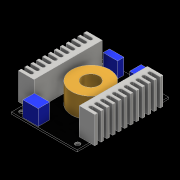
# Autodesk Inventor part: DROK_090483
Saved by Autodesk Inventor 2016 (Build 200138000, 138)
## iProperties
Created: 2016-05-04
Part Number: DROK_090483
Material: Generic
Document SubType Name: Modeling
Designer: CamB
Mass: 20.71 g
Surface Area: 169.365 cm^2
Volume: 20.71 cm^3
Density: 1 g/cm^3
Appearance: Default
Author: CamB
Autodesk Inventor part; units mm, degrees
ref_plane "YZ Plane" through (0, 0, 0) normal (1, 0, 0) x (0, 1, 0)
ref_plane "XZ Plane" through (0, 0, 0) normal (0, 1, 0) x (-1, 0, 0)
sketch "Sketch1" plane through (0, 0, 0) normal (0, 0, 1) x (1, 0, 0)
  line L0 (0, 0) -> (43, 0)
  line L1 (43, 0) -> (43, 60)
  line L2 (43, 60) -> (0, 60)
  line L3 (0, 60) -> (0, 0)
  dimension "d0" = 43
  dimension "d1" = 60
  constraints: 8 end point, 2 parallel, 1 horizontal, 1 perpendicular
  measures "d0" distance of L2.end L1.end
  measures "d1" distance of L1.end L0.end
extrude "PCB" add sketch "Sketch1" along normal blind 1.2
sketch "Sketch2" plane through (0, 0, 1.2) normal (0, 0, 1) x (1, 0, 0)
  line L0 (0, 0) -> (43, 0) projected
  line L1 (43, 0) -> (43, 60) projected
  line L2 (43, 60) -> (0, 60) projected
  line L3 (36.33, 52.83) -> (46.51, 52.83)
  line L4 (46.51, 52.83) -> (46.51, 8.11)
  line L5 (46.51, 8.11) -> (36.33, 8.11)
  line L6 (36.33, 8.11) -> (36.33, 52.83)
  dimension "d4" = 7.17
  dimension "d5" = 8.11
  dimension "d6" = 10.18
  dimension "d8" = 3.51
  constraints: 8 end point, 2 parallel, 1 horizontal, 1 perpendicular
  measures "d4" distance between parallel lines of L2 L3
  measures "d5" distance between parallel lines of L0 L5
  measures "d6" distance between parallel lines of L4 L6
  measures "d8" distance between parallel lines of L1 L4
extrude "Heat Sinks" add sketch "Sketch2" along normal blind 17.7
ref_plane "Work Plane1" through (21.5, 0, 0) normal (-1, 0, 0) x (0, 0, 1)
mirror "Mirror1" about plane through (21.5, 0, 0) normal (-1, 0, 0) of "Heat Sinks"
sketch "Sketch3" plane through (0, 0, 0) normal (0, 0, -1) x (-1, 0, 0)
  line L0 (0, 0) -> (-43, 0) projected
  line L1 (0, 60) -> (0, 0) projected
  line L2 (-43, 60) -> (0, 60) projected
  line L3 (-43, 0) -> (-43, 60) projected
  circle A0 centre (-3.185, 3.585) radius 1.585
  circle A1 centre (-39.815, 3.585) radius 1.585
  circle A2 centre (-39.815, 56.415) radius 1.585
  circle A3 centre (-3.185, 56.415) radius 1.585
  dimension "d11" = 3.17
  dimension "d12" = 3.585
  dimension "d13" = 3.185
  dimension "d14" = 3.17
  dimension "d15" = 3.17
  dimension "d16" = 3.17
  dimension "d17" = 3.185
  dimension "d18" = 3.185
  dimension "d19" = 3.185
  dimension "d20" = 3.585
  dimension "d21" = 3.585
  dimension "d22" = 3.585
  constraints: 4 centre point
  measures "d11" diameter of A0
  measures "d12" distance from line of L0 A0.centre
  measures "d13" distance from line of L1 A0.centre
  measures "d14" diameter of A3
  measures "d15" diameter of A2
  measures "d16" diameter of A1
  measures "d17" distance from line of L3 A1.centre
  measures "d18" distance from line of L3 A2.centre
  measures "d19" distance from line of L1 A3.centre
  measures "d20" distance from line of L2 A3.centre
  measures "d21" distance from line of L2 A2.centre
  measures "d22" distance from line of A1.centre L0
extrude "Extrusion3" cut sketch "Sketch3" against normal blind 2 contours A0 | A1 | A2 | A3
sketch "Sketch4" plane through (0, 0, 1.2) normal (0, 0, 1) x (1, 0, 0)
  line L0 (0, 8.11) -> (0, 0) projected
  line L1 (0, 0) -> (43, 0) projected
  line L2 (43, 52.83) -> (43, 60) projected
  line L3 (43, 60) -> (0, 60) projected
  line L4 (0, 60) -> (0, 52.83) projected
  line L5 (6.46, 53.62) -> (15.96, 53.62)
  line L6 (15.96, 53.62) -> (15.96, 57.84)
  line L7 (15.96, 57.84) -> (6.46, 57.84)
  line L8 (6.46, 57.84) -> (6.46, 53.62)
  line L9 (25.75, 51.79) -> (35.75, 51.79)
  line L10 (35.75, 51.79) -> (35.75, 59.29)
  line L11 (35.75, 59.29) -> (25.75, 59.29)
  line L12 (25.75, 59.29) -> (25.75, 51.79)
  line L13 (7, 8) -> (17, 8)
  line L14 (17, 8) -> (17, 0.5)
  line L15 (17, 0.5) -> (7, 0.5)
  line L16 (7, 0.5) -> (7, 8)
  dimension "d25" = 10
  dimension "d26" = 7.5
  dimension "d27" = 7.5
  dimension "d28" = 10
  dimension "d29" = 9.5
  dimension "d30" = 4.22
  dimension "d31" = 2.16
  dimension "d32" = 6.46
  dimension "d33" = 0.71
  dimension "d34" = 7.25
  dimension "d35" = 0.5
  dimension "d36" = 7
  constraints: 24 end point, 6 parallel, 3 horizontal, 3 perpendicular
  measures "d25" distance of L10.end L11.end
  measures "d26" distance of L9.end L10.end
  measures "d27" distance of L13.end L14.end
  measures "d28" distance of L13.start L13.end
  measures "d29" distance of L6.end L7.end
  measures "d30" distance between parallel lines of L5 L7
  measures "d31" distance between parallel lines of L3 L7
  measures "d32" distance between parallel lines of L4 L8
  measures "d33" distance between parallel lines of L3 L11
  measures "d34" distance between parallel lines of L2 L10
  measures "d35" distance between parallel lines of L1 L15
  measures "d36" distance between parallel lines of L0 L16
extrude "Extrusion4" add sketch "Sketch4" along normal blind 10.18
sketch "Sketch5" plane through (0, 0, 1.2) normal (0, 0, 1) x (1, 0, 0)
  line L0 (36.33, 8.11) -> (36.33, 52.83) projected
  line L1 (43, 60) -> (0, 60) projected
  circle A0 centre (21.5, 30.47) radius 12.5
  circle A1 centre (21.5, 30.47) radius 5.45
  point P0 (21.5, 60)
  point P1 (36.33, 30.47)
  dimension "d39" = 25
  dimension "d40" = 10.9
  constraints: 2 centre point, 2 midpoint, 1 horizontal alignment, 1 vertical alignment
  measures "d39" diameter of A0
  measures "d40" diameter of A1
extrude "Extrusion5" add sketch "Sketch5" along normal blind 13.34
sketch "Sketch6" plane through (0, 0, 18.9) normal (0, 0, 1) x (1, 0, 0)
  line L0 (46.51, 52.83) -> (36.33, 52.83) projected
  line L1 (46.51, 8.11) -> (46.51, 52.83) projected
  line L2 (51.51, 50.93) -> (40.885, 50.93)
  line L3 (39.76, 49.805) -> (39.76, 49.805)
  line L4 (40.885, 48.68) -> (51.51, 48.68)
  line L5 (51.51, 48.68) -> (51.51, 50.93)
  arc A0 (40.885, 50.93) -> (39.76, 49.805) centre (40.885, 49.805) ccw
  arc A1 (39.76, 49.805) -> (40.885, 48.68) centre (40.885, 49.805) ccw
  line L6 (51.51, 47.06) -> (40.885, 47.06)
  line L7 (39.76, 45.935) -> (39.76, 45.935)
  line L8 (40.885, 44.81) -> (51.51, 44.81)
  line L9 (51.51, 44.81) -> (51.51, 47.06)
  arc A2 (40.885, 47.06) -> (39.76, 45.935) centre (40.885, 45.935) ccw
  arc A3 (39.76, 45.935) -> (40.885, 44.81) centre (40.885, 45.935) ccw
  line L10 (51.51, 43.19) -> (40.885, 43.19)
  line L11 (39.76, 42.065) -> (39.76, 42.065)
  line L12 (40.885, 40.94) -> (51.51, 40.94)
  line L13 (51.51, 40.94) -> (51.51, 43.19)
  arc A4 (40.885, 43.19) -> (39.76, 42.065) centre (40.885, 42.065) ccw
  arc A5 (39.76, 42.065) -> (40.885, 40.94) centre (40.885, 42.065) ccw
  line L14 (51.51, 39.32) -> (40.885, 39.32)
  line L15 (39.76, 38.195) -> (39.76, 38.195)
  line L16 (40.885, 37.07) -> (51.51, 37.07)
  line L17 (51.51, 37.07) -> (51.51, 39.32)
  arc A6 (40.885, 39.32) -> (39.76, 38.195) centre (40.885, 38.195) ccw
  arc A7 (39.76, 38.195) -> (40.885, 37.07) centre (40.885, 38.195) ccw
  line L18 (51.51, 35.45) -> (40.885, 35.45)
  line L19 (39.76, 34.325) -> (39.76, 34.325)
  line L20 (40.885, 33.2) -> (51.51, 33.2)
  line L21 (51.51, 33.2) -> (51.51, 35.45)
  arc A8 (40.885, 35.45) -> (39.76, 34.325) centre (40.885, 34.325) ccw
  arc A9 (39.76, 34.325) -> (40.885, 33.2) centre (40.885, 34.325) ccw
  line L22 (51.51, 31.58) -> (40.885, 31.58)
  line L23 (39.76, 30.455) -> (39.76, 30.455)
  line L24 (40.885, 29.33) -> (51.51, 29.33)
  line L25 (51.51, 29.33) -> (51.51, 31.58)
  arc A10 (40.885, 31.58) -> (39.76, 30.455) centre (40.885, 30.455) ccw
  arc A11 (39.76, 30.455) -> (40.885, 29.33) centre (40.885, 30.455) ccw
  line L26 (51.51, 27.71) -> (40.885, 27.71)
  line L27 (39.76, 26.585) -> (39.76, 26.585)
  line L28 (40.885, 25.46) -> (51.51, 25.46)
  line L29 (51.51, 25.46) -> (51.51, 27.71)
  arc A12 (40.885, 27.71) -> (39.76, 26.585) centre (40.885, 26.585) ccw
  arc A13 (39.76, 26.585) -> (40.885, 25.46) centre (40.885, 26.585) ccw
  line L30 (51.51, 23.84) -> (40.885, 23.84)
  line L31 (39.76, 22.715) -> (39.76, 22.715)
  line L32 (40.885, 21.59) -> (51.51, 21.59)
  line L33 (51.51, 21.59) -> (51.51, 23.84)
  arc A14 (40.885, 23.84) -> (39.76, 22.715) centre (40.885, 22.715) ccw
  arc A15 (39.76, 22.715) -> (40.885, 21.59) centre (40.885, 22.715) ccw
  line L34 (51.51, 19.97) -> (40.885, 19.97)
  line L35 (39.76, 18.845) -> (39.76, 18.845)
  line L36 (40.885, 17.72) -> (51.51, 17.72)
  line L37 (51.51, 17.72) -> (51.51, 19.97)
  arc A16 (40.885, 19.97) -> (39.76, 18.845) centre (40.885, 18.845) ccw
  arc A17 (39.76, 18.845) -> (40.885, 17.72) centre (40.885, 18.845) ccw
  line L38 (51.51, 16.1) -> (40.885, 16.1)
  line L39 (39.76, 14.975) -> (39.76, 14.975)
  line L40 (40.885, 13.85) -> (51.51, 13.85)
  line L41 (51.51, 13.85) -> (51.51, 16.1)
  arc A18 (40.885, 16.1) -> (39.76, 14.975) centre (40.885, 14.975) ccw
  arc A19 (39.76, 14.975) -> (40.885, 13.85) centre (40.885, 14.975) ccw
  line L42 (51.51, 12.23) -> (40.885, 12.23)
  line L43 (39.76, 11.105) -> (39.76, 11.105)
  line L44 (40.885, 9.98) -> (51.51, 9.98)
  line L45 (51.51, 9.98) -> (51.51, 12.23)
  arc A20 (40.885, 12.23) -> (39.76, 11.105) centre (40.885, 11.105) ccw
  arc A21 (39.76, 11.105) -> (40.885, 9.98) centre (40.885, 11.105) ccw
  point P0 (36.33, 8.11)
  point P1 (0, 0)
  dimension "d43" = 5
  dimension "d44" = 6.75
  dimension "d45" = 2.25
  dimension "d46" = 1.9
  dimension "d54" = 44.72
  dimension "d56" = 1.125
  dimension "d57" = 1.125
  dimension "d60" = 3.87
  constraints: 88 end point, 44 point on circle, 22 centre point, 4 tangent, 2 parallel, 1 horizontal, 1 perpendicular, 1 vertical, 140 other
  measures "d43" distance between parallel lines of L1 L5
  measures "d44" distance between parallel lines of L1 L3
  measures "d45" distance of L4.end L2.start
  measures "d46" distance between parallel lines of L0 L2
  measures "d54" distance of L0.end point (36.33, 8.11)
  measures "d56" radius of A0
  measures "d57" radius of A1
  measures "d60" distance of L2.start L6.start
extrude "Extrusion6" cut sketch "Sketch6" against normal up to surface (17.7 mm away)
mirror "Mirror2" about plane through (21.5, 0, 0) normal (-1, 0, 0) of "Extrusion6"
equation "\"d14\" = d11"
equation "\"d15\" = d14"
equation "\"d16\" = d15"
equation "\"d17\" = d13"
equation "\"d18\" = d17"
equation "\"d19\" = d18"
equation "\"d20\" = d12"
equation "\"d21\" = d20"
equation "\"d22\" = d12"
equation "\"d27\" = d26"
equation "\"d28\" = d25"
equation "\"d56\" = 0.5 * d45"
equation "\"d57\" = d56"
body "Solid1"
